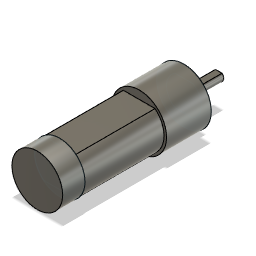
IG220019X00015R v1 (Autodesk Fusion 360 design; units mm, degrees)
Autodesk Fusion 360 part; units mm, degrees
note: some values were not read from the file. Set by a fixed rule: which sketch regions a step uses.
sketch "スケッチ1" plane through (0, 0, 0) normal (0, 0, 1) x (1, 0, 0)
  circle A0 centre (0, 0) radius 11
  dimension "d1" = 22
  constraint coincident A0.centre origin
  measures "d1" diameter of A0
extrude "押し出し1" add sketch "スケッチ1" along normal blind 18
sketch "スケッチ2" plane through (0, 0, 18) normal (0, 0, 1) x (1, 0, 0)
  circle A0 centre (0, 0) radius 11
  circle A1 centre (0, 0) radius 10
  line L0 (-7, -7.7) -> (7, -7.7)
  line L1 (7, -7.7) -> (7, 7.7)
  line L2 (7, 7.7) -> (-7, 7.7)
  line L3 (-7, 7.7) -> (-7, -7.7)
  line L4 (-7, -7.7) -> (7, 7.7) construction
  line L5 (7, -7.7) -> (-7, 7.7) construction
  dimension "d4" = 20
  dimension "d5" = 14
  dimension "d6" = 15.4
  constraint concentric A0 A1
  constraint horizontal L0
  constraint perpendicular L0 L1
  constraint parallel L0 L2
  constraint parallel L1 L3
  constraint coincident L4 A0.centre
  constraint coincident L5 A0.centre
  constraint coincident A0.centre A1.centre
  measures "d4" diameter of A1
  measures "d5" distance of L1.end L2.end
  measures "d6" distance of L0.end L1.end
sketch "スケッチ3" plane through (0, 0, 18) normal (0, 0, 1) x (1, 0, 0)
extrude "押し出し2" add sketch "スケッチ2" along normal blind 32 contours A1 L1 | A1 L0 L1 L2 L3 | A1 L3
sketch "スケッチ4" plane through (0, 0, 50) normal (0, 0, 1) x (1, 0, 0)
  arc A0 (6.3804, -7.7) -> (6.3804, 7.7) centre (0, 0) ccw
  line L0 (6.3804, 7.7) -> (-6.3804, 7.7)
  arc A1 (-6.3804, 7.7) -> (-6.3804, -7.7) centre (0, 0) ccw
  line L1 (-6.3804, -7.7) -> (6.3804, -7.7)
  circle A2 centre (0, 0) radius 10.2
  dimension "d9" = 20.4
  constraint coincident A0.centre A1.centre
  measures "d9" diameter of A2
extrude "押し出し3" add sketch "スケッチ4" along normal blind 9 contours A0 L0 A1 L1 | A2
sketch "スケッチ5" plane through (0, 0, 0) normal (0, 0, -1) x (-1, 0, 0)
  circle A0 centre (0, 0) radius 11
  circle A1 centre (0, 0) radius 6.9
  line L0 (6, 3.45) -> (-6, 3.45)
  line L1 (-6, 3.45) -> (-6, -3.45)
  line L2 (-6, -3.45) -> (6, -3.45)
  line L3 (6, -3.45) -> (6, 3.45)
  line L4 (6, 3.45) -> (-6, -3.45) construction
  line L5 (-6, 3.45) -> (6, -3.45) construction
  dimension "d12" = 13.8
  dimension "d13" = 12
  dimension "d14" = 6.9
  constraint concentric A0 A1
  constraint horizontal L0
  constraint perpendicular L0 L1
  constraint parallel L0 L2
  constraint parallel L1 L3
  constraint coincident L4 A0.centre
  constraint coincident L5 A0.centre
  constraint coincident A0.centre A1.centre
  measures "d12" diameter of A1
  measures "d13" distance of L1.end L2.end
  measures "d14" distance of L0.end L1.end
extrude "押し出し4" add sketch "スケッチ5" along normal blind 2 contours A1 L3 | A1 L0 L1 L2 L3 | A1 L1
sketch "スケッチ6" plane through (0, 0, -2) normal (0, 0, -1) x (-1, 0, 0)
  arc A0 (-5.9756, 3.45) -> (-5.9756, -3.45) centre (0, 0) ccw
  line L0 (-5.9756, -3.45) -> (5.9756, -3.45)
  arc A1 (5.9756, -3.45) -> (5.9756, 3.45) centre (0, 0) ccw
  line L1 (5.9756, 3.45) -> (-5.9756, 3.45)
  circle A2 centre (0, 0) radius 2
  dimension "d17" = 4
  constraint coincident A0.centre A1.centre
  measures "d17" diameter of A2
extrude "押し出し5" add sketch "スケッチ6" along normal blind 4 contours A2
sketch "スケッチ8" plane through (0, 0, 18) normal (0, 0, 1) x (1, 0, 0)
  circle A0 centre (0, 0) radius 2
  dimension "d22" = 4
  constraint coincident A0.centre origin
  measures "d22" diameter of A0
extrude "押し出し6" add 1 faces at (-0.637, 0.1965, -6) along direction (0, 0, -1) blind 8
sketch "スケッチ9" plane through (0, 0, -14) normal (0, 0, -1) x (-1, 0, 0)
  circle A0 centre (0, 0) radius 2
  line L0 (0, 2) -> (-2.3, 2)
  line L1 (-2.3, 2) -> (-2.3, 1.5)
  line L2 (-2.3, 1.5) -> (0, 1.5)
  line L3 (0, 1.5) -> (0, 2)
  circle A1 centre (0, 0) radius 2
  line L4 (0, 1.5) -> (1.7491, 1.5)
  line L5 (1.7491, 1.5) -> (1.7491, 2)
  line L6 (1.7491, 2) -> (0, 2)
  line L7 (0, 2) -> (0, 1.5)
  constraint horizontal L0
  constraint vertical L1
  constraint horizontal L2
  constraint vertical L3
  constraint coincident A0 L0.start
  constraint coincident A0.centre A1.centre
  constraint horizontal L4
  constraint vertical L5
  constraint horizontal L6
  constraint vertical L7
extrude "押し出し7" cut sketch "スケッチ9" against normal blind 8 contours A0 L3 A1 L4 L7 | A0 L2 L3 A1 L7
sketch "スケッチ10" plane through (0, 0, 0) normal (0, 0, -1) x (-1, 0, 0)
  line L0 (-5.9756, 3.45) -> (5.9756, 3.45)
  arc A0 (5.9756, -3.45) -> (5.9756, 3.45) centre (0, 0) ccw
  line L1 (5.9756, -3.45) -> (-5.9756, -3.45)
  arc A1 (-5.9756, 3.45) -> (-5.9756, -3.45) centre (0, 0) ccw
  circle A2 centre (0, 0) radius 11
  circle A3 centre (0, 0) radius 7
  line L2 (7, 6) -> (-7, 6)
  line L3 (-7, 6) -> (-7, -6)
  line L4 (-7, -6) -> (7, -6)
  line L5 (7, -6) -> (7, 6)
  line L6 (7, 6) -> (-7, -6) construction
  line L7 (-7, 6) -> (7, -6) construction
  dimension "d27" = 14
  dimension "d28" = 14
  dimension "d29" = 12
  constraint concentric A0 A3
  constraint horizontal L2
  constraint perpendicular L2 L3
  constraint parallel L2 L4
  constraint parallel L3 L5
  constraint coincident L6 A0.centre
  constraint coincident L7 A0.centre
  constraint coincident A0.centre A1.centre
  measures "d27" diameter of A3
  measures "d28" distance of L3.end L4.end
  measures "d29" distance of L2.end L3.end
extrude "押し出し8" add sketch "スケッチ10" along normal blind 2 contours A3 L2 L4
sketch "スケッチ11" plane through (0, 0, 0) normal (0, 0, -1) x (-1, 0, 0)
  line L0 (-3.6056, 6) -> (3.6056, 6)
  arc A0 (3.6056, -6) -> (3.6056, 6) centre (0, 0) ccw
  line L1 (3.6056, -6) -> (-3.6056, -6)
  arc A1 (-3.6056, 6) -> (-3.6056, -6) centre (0, 0) ccw
  circle A2 centre (0, 0) radius 11
sketch "スケッチ12" plane through (0, 0, 0) normal (0, 0, -1) x (-1, 0, 0)
  line L0 (11, 0) -> (-11, 0)
  line L1 (-11, 0) -> (-11, -11)
  line L2 (-11, -11) -> (0, 0)
  line L3 (0, 0) -> (7.7782, 7.7782)
  circle A0 centre (0, 0) radius 9
  circle A1 centre (-6.364, -6.364) radius 1
  line L4 (0, 1.75) -> (0, 22.5)
  circle A2 centre (6.364, -6.364) radius 1
  circle A3 centre (6.364, 6.364) radius 1
  circle A4 centre (-6.364, 6.364) radius 1
  dimension "d32" = 11
  dimension "d33" = 180
  dimension "d34" = 11
  dimension "d35" = 18
  dimension "d36" = 2
  constraint horizontal L0
  constraint perpendicular L0 L1
  constraint coincident L2.end L3.start
  constraint coincident A0 A1.centre
  constraint coincident L2 A1.centre
  constraint symmetric A1 L4 A2
  constraint symmetric L0 A1 A4
  constraint symmetric L0 A2 A3
  measures "d32" distance of L0.end L1.end
  measures "d33" angle of L2 L3
  measures "d34" distance of L2.end L3.end
  measures "d35" diameter of A0
  measures "d36" diameter of A1
extrude "押し出し9" cut sketch "スケッチ12" against normal blind 4 contours L3 A0 A3 | L3 A0 A3 | A0 A2 | A0 A2 | L2 A0 A1 | L2 A0 A1 | L3 A0 A3 | L3 A0 A3 | A0 A4 | A0 A4 | L2 A0 A1 | L2 A0 A1
sketch "スケッチ14" plane through (0, 0, 50) normal (0, 0, -1) x (-1, 0, 0)
  circle A0 centre (0, 0) radius 10.2
  line L0 (6.3804, -7.7) -> (-6.3804, -7.7)
  arc A1 (-6.3804, 7.7) -> (-6.3804, -7.7) centre (0, 0) ccw
  line L1 (-6.3804, 7.7) -> (6.3804, 7.7)
  arc A2 (6.3804, -7.7) -> (6.3804, 7.7) centre (0, 0) ccw
